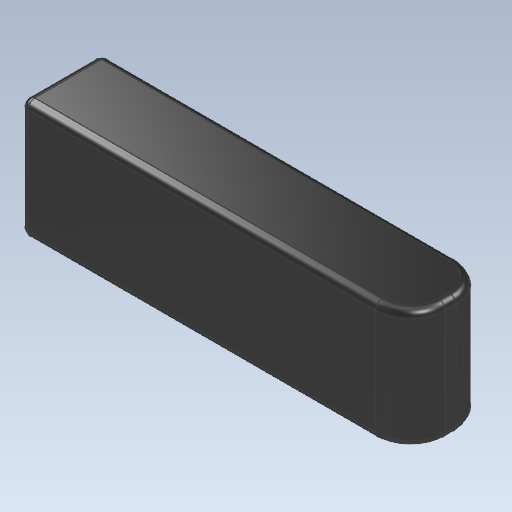
# Autodesk Inventor part: HP-G830C2800S3
Saved by Autodesk Inventor 2020.4 (Build 244396000, 396)
## iProperties
Created: 2022-01-01
Part Number: HP-G830C2800S3
Material: 一般
Catalog Web Link: https://hyperion-world.com/en/g8-3s-2800mah-si-graphene-lightweight-lipo-30c-4-35-4-2v
Document SubType Name: Modeling
Designer: Masato Kubotera
Mass: 181 g
Surface Area: 133.325 cm^2
Volume: 84.8467 cm^3
Density: 2.08521 g/cm^3
Appearance: 光沢 - 黒
Description: 既製品
Author: Masato Kubotera
Autodesk Inventor part; units mm, degrees
ref_plane "YZ Plane" through (0, 0, 0) normal (1, 0, 0) x (0, 1, 0)
ref_plane "XZ Plane" through (0, 0, 0) normal (0, 1, 0) x (-1, 0, 0)
ref_plane "XY Plane" through (0, 0, 0) normal (0, 0, 1) x (1, 0, 0)
sketch "スケッチ1" plane through (0, 0, 0) normal (0, 0, 1) x (1, 0, 0)
  line L0 (-55.5, 17) -> (55.5, 17)
  line L1 (55.5, 17) -> (55.5, -17)
  line L2 (55.5, -17) -> (-55.5, -17)
  line L3 (-55.5, -17) -> (-55.5, 17)
  line L4 (-55.5, 17) -> (55.5, -17) construction
  line L5 (55.5, 17) -> (-55.5, -17) construction
  point P0 (0, 0)
  dimension "d0" = 111
  dimension "d1" = 34
  constraints: 12 end point, 2 midpoint, 2 parallel, 1 horizontal, 1 perpendicular
  measures "d0" distance of L1.end L2.end
  measures "d1" distance of L0.end L1.end
extrude "押し出し1" add sketch "スケッチ1" along normal blind 23
fillet "フィレット1" radius 10 2 edges at (55.5, 0, 23) (55.5, 0, 0)
fillet "フィレット2" radius 2 14 edges at (-55.5, 0, 23) (-55.5, 17, 11.5) (-55.5, 0, 0) (-55.5, -17, 11.5) (52.5711, 17, 20.0711) (55.5, 17, 11.5) (52.5711, 17, 2.9289) (-5, 17, 0) (-5, 17, 23) (52.5711, -17, 20.0711) (55.5, -17, 11.5) (52.5711, -17, 2.9289) (-5, -17, 0) (-5, -17, 23)
